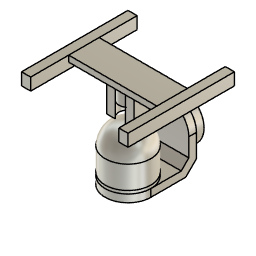
5 Axis CNC Linkage Ideation (Autodesk Fusion 360 design; units mm, degrees)
Autodesk Fusion 360 part; units mm, degrees
note: some values were not read from the file. Chosen so that the rebuilt part matches the saved one: which bodies a step acts on.
sketch "Sketch1" plane through (0, 0, 0) normal (0, 0, 1) x (1, 0, 0)
  circle A0 centre (0, 0) radius 150
  line L0 (-150, 0) -> (150, 0) construction
  line L1 (150, 0) -> (150, 250)
  line L2 (150, 250) -> (-150, 250)
  line L3 (-150, 250) -> (-150, 0)
  line L4 (-150, 250) -> (150, 250)
  line L5 (150, 250) -> (150, 300)
  line L6 (150, 300) -> (-150, 300)
  line L7 (-150, 300) -> (-150, 250)
  dimension "d7" = 300
  dimension "d8" = 250
  dimension "d9" = 50
  constraint coincident A0.centre origin
  constraint horizontal L0
  constraint vertical L1
  constraint horizontal L2
  constraint vertical L3
  constraint coincident A0 L0.start
  constraint coincident A0 L0.end
  constraint coincident A0.centre L0
  constraint horizontal L4
  constraint vertical L5
  constraint horizontal L6
  constraint vertical L7
  constraint collinear L1 L5
  measures "d7" diameter of A0
  measures "d8" distance of L0.end L1.end
  measures "d9" distance of L2.end L6.end
extrude "Extrude6" add sketch "Sketch1" along normal mid plane 300 contours A0 makes body 1
extrude "Extrude7" add sketch "Sketch1" against normal blind 20 from surface at -150 separate body contours A0 makes body 2
fillet "Fillet3" radius 150 1 edges at (-139.8491, -54.2423, 150) on bodies 1
extrude "Extrude8" add sketch "Sketch1" against normal blind 50 from surface at -170 separate body makes body 3
extrude "Extrude9" add sketch "Sketch1" along normal blind 20 from surface at -170 contours L2 L4 L5 L6 L7 bodies 3
extrude "Extrude10" add sketch "Sketch1" along normal mid plane 300 separate body contours L2 L4 L5 L6 L7 makes body 4
extrude "Extrude11" add 1 faces at (-50, 300, 50) along direction (0, 1, 0) blind 50 separate body on bodies 4 makes body 5
combine "Combine1" operation add target body 3 tool bodies 4
fillet "Fillet2" radius 150 6 edges at (150, 275, 150) (-150, 275, 150) (150, 325, 150) (-150, 325, 150) (-150, 325, -150) (150, 325, -150) on bodies 3 5
chamfer "Chamfer1" distance 50 angle 45 1 edges at (0, 250, -170) on bodies 3
chamfer "Chamfer1" distance 70 angle 45 1 edges at (0, 300, -220) on bodies 3
sketch "Sketch2" plane through (0, 0, 0) normal (1, 0, 0) x (0, 1, 0)
  line L0 (-60, 420) -> (60, 420)
  line L1 (60, 420) -> (60, 380)
  line L2 (60, 380) -> (-60, 380)
  line L3 (-60, 380) -> (-60, 420)
  line L4 (-60, 420) -> (60, 380) construction
  line L5 (60, 420) -> (-60, 380) construction
  line L6 (0, 0) -> (0, 400)
  line L7 (60, 380) -> (-60, 380)
  line L8 (-60, 380) -> (-60, 260)
  line L9 (-60, 260) -> (60, 260)
  line L10 (60, 260) -> (60, 380)
  line L11 (-350, 420) -> (350, 420)
  line L12 (350, 420) -> (350, 380)
  line L13 (350, 380) -> (-350, 380)
  line L14 (-350, 380) -> (-350, 420)
  line L15 (-350, 420) -> (350, 380) construction
  line L16 (350, 420) -> (-350, 380) construction
  line L17 (-5, 260) -> (5, 260)
  line L18 (5, 260) -> (5, 160)
  line L19 (5, 160) -> (-5, 160)
  line L20 (-5, 160) -> (-5, 260)
  line L21 (-5, 260) -> (5, 160) construction
  line L22 (5, 260) -> (-5, 160) construction
  line L23 (-50, 380) -> (50, 380)
  line L24 (50, 380) -> (50, 260)
  line L25 (50, 260) -> (-50, 260)
  line L26 (-50, 260) -> (-50, 380)
  line L27 (-50, 380) -> (50, 260) construction
  line L28 (50, 380) -> (-50, 260) construction
  point P0 (0, 400)
  point P1 (0, 400)
  point P2 (0, 210)
  point P3 (0, 320)
  dimension "d43" = 120
  dimension "d44" = 40
  dimension "d45" = 400
  dimension "d46" = 120
  dimension "d47" = 700
  dimension "d48" = 40
  dimension "d56" = 10
  dimension "d57" = 100
  dimension "d58" = 100
  constraint horizontal L0
  constraint perpendicular L0 L1
  constraint parallel L0 L2
  constraint parallel L1 L3
  constraint coincident L4 P1
  constraint coincident L5 P1
  constraint coincident L6.start origin
  constraint perpendicular L2 L6
  constraint coincident P1 P0
  constraint horizontal L7
  constraint vertical L8
  constraint horizontal L9
  constraint vertical L10
  constraint collinear L3 L8
  constraint horizontal L11
  constraint perpendicular L11 L12
  constraint parallel L11 L13
  constraint parallel L12 L14
  constraint coincident L15 P1
  constraint coincident L16 P1
  constraint horizontal L17
  constraint perpendicular L17 L18
  constraint parallel L17 L19
  constraint parallel L18 L20
  constraint coincident L21 P2
  constraint coincident L22 P2
  constraint coincident L6 P2
  constraint collinear L9 L17
  constraint horizontal L23
  constraint perpendicular L23 L24
  constraint parallel L23 L25
  constraint parallel L24 L26
  constraint coincident L27 P3
  constraint coincident L28 P3
  constraint coincident L6 P3
  constraint collinear L9 L25
  constraint collinear L2 L23
  measures "d43" distance of L1.end L2.end
  measures "d44" distance of L0.end L1.end
  measures "d45" distance of L6.start P1
  measures "d46" distance of L1.end L9.end
  measures "d47" distance of L12.end L13.end
  measures "d48" distance of L11.end L12.end
  measures "d56" distance of L18.end L19.end
  measures "d57" distance of L17.end L18.end
  measures "d58" distance of L24.end L25.end
extrude "Extrude12" add sketch "Sketch2" along normal mid plane 700 separate body contours L0 L1 L2 L3 L7 L11 L13 L23 | L3 L11 L13 L14 | L1 L11 L12 L13 makes body 6
extrude "Extrude13" cut sketch "Sketch2" along normal mid plane 580 contours L0 L1 L2 L3 L7 L11 L13 L23 | L3 L11 L13 L14 | L1 L11 L12 L13 bodies 6 makes body 7 at (330, -116.6667, 420)
extrude "Extrude14" add sketch "Sketch2" along normal mid plane 580 separate body contours L0 L1 L2 L3 L7 L11 L13 L23 makes body 8
revolve "Revolve1" add sketch "Sketch2" angle 360 about axis through (0, 0, 0) along (0, 0, 1) separate body contours L2 L7 L9 L10 L13 L24 | L2 L6 L7 L9 L13 L17 L23 L24 L25 | L6 L9 L17 L18 L19 L25 makes body 9
extrude "Extrude15" add sketch "Sketch2" along normal mid plane 180 separate body contours L2 L6 L7 L9 L13 L17 L23 L25 L26 | L2 L6 L7 L9 L13 L17 L23 L24 L25 makes body 10
combine "Combine2" operation cut target body 10 tool bodies 9 keep tools makes body 11 at (35.4744, 48.3897, 340)
extrude "Extrude17" add 2 faces at (80, 0, 260) (-80, 0, 260) along direction (0, 0, -1) blind 100 on bodies 10 11 bodies 11 10
move_face "OffsetFaces1" offset 40 1 faces at (96.6667, 60, 406.6667) on bodies 8
move_face "OffsetFaces2" offset 40 1 faces at (96.6667, -60, 393.3333) on bodies 8
move_face "OffsetFaces3" offset 40 2 faces at (-310, 116.6667, 380) (330, 116.6667, 380) on bodies 6 7
sketch "Sketch3" plane through (0, 0, 0) normal (1, 0, 0) x (0, 1, 0)
  line L0 (400, 500) -> (-400, 500)
  line L1 (-400, 500) -> (-400, -300)
  line L2 (-400, -300) -> (400, -300)
  line L3 (400, -300) -> (400, 500)
  line L4 (400, 500) -> (-400, -300) construction
  line L5 (-400, 500) -> (400, -300) construction
  point P0 (0, 100)
  dimension "d69" = 800
  dimension "d70" = 800
  constraint horizontal L0
  constraint perpendicular L0 L1
  constraint parallel L0 L2
  constraint parallel L1 L3
  constraint coincident L4 P0
  constraint coincident L5 P0
  measures "d69" distance of L1.end L2.end
  measures "d70" distance of L0.end L1.end
extrude "Extrude18" add sketch "Sketch3" along normal mid plane 800 separate body makes body 12
hidden bodies 12
named bodies: "Fabricatable Volume", "Work Table", "Rotary Arm", "Rotation Linkage", "Gantry Y A", "Gantry Y B", "Gantry X", "Spindle", "Z A", "Z B", "Total Volume"
